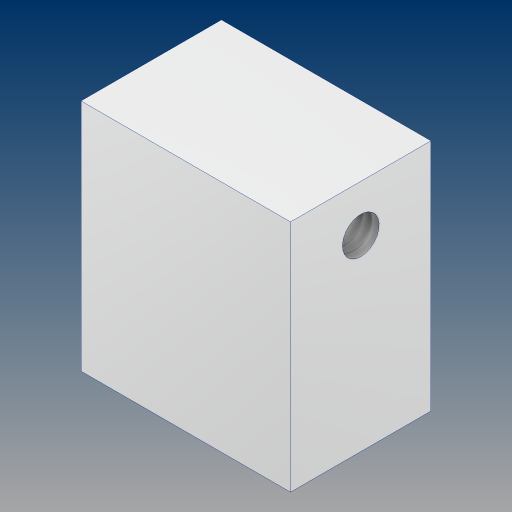
# Autodesk Inventor part: Intake Pivot Billet
Saved by Autodesk Inventor 2024.3 (Build 283343000, 343)
## iProperties
Created: 2024-08-02
Part Number: Intake Pivot Billet
Material: Aluminum 6061
Document SubType Name: Modeling
Designer: Kenji
Density: 2.7 g/cm^3
Appearance: Aluminum - Flat
Author: Kenji
Autodesk Inventor part; units mm, degrees
ref_plane "YZ Plane" through (0, 0, 0) normal (1, 0, 0) x (0, 1, 0)
ref_plane "XZ Plane" through (0, 0, 0) normal (0, 1, 0) x (-1, 0, 0)
ref_plane "XY Plane" through (0, 0, 0) normal (0, 0, 1) x (1, 0, 0)
sketch "Sketch1" plane through (0, 0, 0) normal (1, 0, 0) x (0, 1, 0)
  line L0 (0, 0) -> (31.75, 0)
  line L1 (31.75, 0) -> (31.75, -19.05)
  line L2 (31.75, -19.05) -> (0, -19.05)
  line L3 (0, -19.05) -> (0, 0)
  circle A0 centre (25.4, -9.525) radius 3.2512 construction
  dimension "d0" = 31.75
  dimension "d1" = 19.05
  dimension "d2" = 6.5024
  dimension "d3" = 6.35
  dimension "d4" = 9.525
  constraints: 8 end point, 2 parallel, 1 centre point, 1 coincident, 1 horizontal, 1 perpendicular
  measures "d0" distance of L1.end L2.end
  measures "d1" distance of L0.end L1.end
  measures "d2" diameter of A0
  measures "d3" distance from line of L1 A0.centre
  measures "d4" distance from line of L0 A0.centre
extrude "Extrusion1" add sketch "Sketch1" along normal blind 28.4226
hole "Hole1" at (0, 25.4, -9.525) at (0, 25.4, -9.525) direction (1, 0, 0) diameter 4.9784 end through all thread size "1/4-20 UNC" class "2B" standard "ANSI Unified Screw Threads"
sketch "Sketch2" plane through (0, 0, -19.05) normal (0, -1, 0) x (1, 0, 0)
  line L0 (0, 19.05) -> (0, 0) projected
  line L1 (0, 0) -> (28.4226, 0) projected
  line L2 (28.4226, 19.05) -> (28.4226, 0) projected
  line L3 (0, 19.05) -> (28.4226, 19.05) projected
  line L4 (28.4226, 2.307) -> (7.7724, 2.307) construction
  point P0 (18.3515, 9.525)
  dimension "d14" = 20.6502
  dimension "d15" = 10.0711
  dimension "d16" = 9.525
  constraints: 2 end point, 1 parallel, 1 point on line
  measures "d14" distance of L4.start L4.end
  measures "d15" horizontal distance of L4.start point (18.351, 9.525)
  measures "d16" distance from line of point (18.351, 9.525) L1
hole "Hole2" at (18.3515, 0, -9.525) direction (0, 1, 0) diameter 4.9784 depth 19.05 thread size "1/4-20 UNC" class "2B" standard "ANSI Unified Screw Threads"
body "Solid1"
